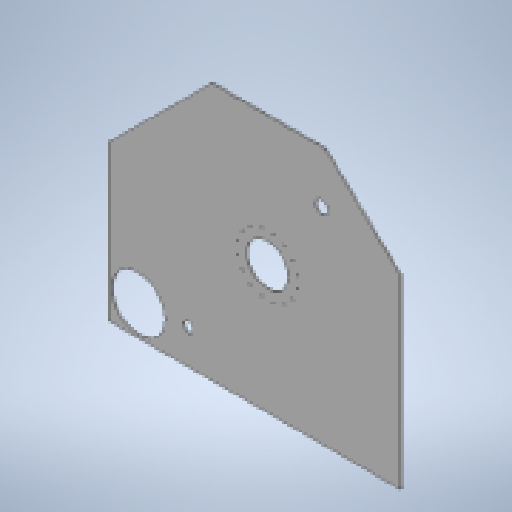
# Autodesk Inventor part: Left wall v2.0
Saved by Autodesk Inventor 2026.3 (Build 303398000, 398)
## iProperties
Created: 2023-08-31
Part Number: Left wall v2.0
Material: Generic
Document SubType Name: Sheet Metal
Designer: admin
Density: 1 g/cm^3
Appearance: Default
Flat Pattern Width: 191 cm
Flat Pattern Length: 217 cm
Flat Pattern Area: 41447 cm^2
Sheet Metal Rule: Default
Sheet Metal Width: 1910,000 mm
Sheet Metal Length: 2170,000 mm
Sheet Metal Area: 4144700,000 mm^2
Stock Number: ДМФ 013 Стенка Нос
Author: admin
Autodesk Inventor part; units mm, degrees
ref_plane "YZ Plane" through (0, 0, 0) normal (1, 0, 0) x (0, 1, 0)
ref_plane "XZ Plane" through (0, 0, 0) normal (0, 1, 0) x (-1, 0, 0)
ref_plane "XY Plane" through (0, 0, 0) normal (0, 0, 1) x (1, 0, 0)
sketch "Sketch1" plane through (0, 0, 0) normal (0, 0, 1) x (1, 0, 0)
  line L0 (519.5155, 1910) -> (-320.4845, 1910)
  line L1 (-320.4845, 1910) -> (-1085, 1150)
  line L2 (-1085, 0) -> (-1085, 1150)
  line L3 (1085, 0) -> (1085, 1372.7595)
  line L4 (519.5155, 1910) -> (1085, 1372.7595)
  line L5 (1085, 0) -> (-1085, 0)
  circle A0 centre (-865, 220) radius 200.5
  circle A1 centre (-493, 255) radius 38
  circle A2 centre (120, 955) radius 700 construction
  line L6 (499.31, 1277) -> (499.31, 1910) construction
  circle A3 centre (499.31, 1543.323) radius 30
  line L7 (1085, 955) -> (325, 955) construction
  circle A4 centre (120, 955) radius 205
  line L8 (120, 0) -> (120, 750) construction
  circle A5 centre (120, 955) radius 225 construction
  circle A6 centre (163.8953, 1175.6767) radius 6
  line L9 (120, 955) -> (120, 1180) construction
  line L10 (163.8953, 1175.6767) -> (120, 955) construction
  circle A7 centre (76.1047, 1175.6767) radius 6
  circle A8 centre (-5.0033, 1142.0807) radius 6
  circle A9 centre (-67.0807, 1080.0033) radius 6
  circle A10 centre (-100.6767, 998.8953) radius 6
  circle A11 centre (-100.6767, 911.1047) radius 6
  circle A12 centre (-67.0807, 829.9967) radius 6
  circle A13 centre (-5.0033, 767.9193) radius 6
  circle A14 centre (76.1047, 734.3233) radius 6
  circle A15 centre (163.8953, 734.3233) radius 6
  circle A16 centre (245.0033, 767.9193) radius 6
  circle A17 centre (307.0807, 829.9967) radius 6
  circle A18 centre (340.6767, 911.1047) radius 6
  circle A19 centre (340.6767, 998.8953) radius 6
  circle A20 centre (307.0807, 1080.0033) radius 6
  circle A21 centre (245.0033, 1142.0807) radius 6
  circle A22 centre (120, 955) radius 670 construction
  point P0 (0, 0)
  dimension "d69" = 1400
  dimension "d1" = 840
  dimension "d3" = 1150
  dimension "d14" = 76
  dimension "d15" = 1910
  dimension "d16" = 255
  dimension "d17" = 220
  dimension "d18" = 401
  dimension "d19" = 220
  dimension "d33" = 2170
  dimension "d49" = 372
  dimension "d51" = 780
  dimension "d52" = 1078
  dimension "d70" = 1584.31
  dimension "d71" = 60
  dimension "d74" = 760
  dimension "d75" = 410
  dimension "d76" = 750
  dimension "d77" = 450
  dimension "d78" = 12
  dimension "d79" = 11.25
  dimension "d82" = 360
  dimension "d84" = 465
  constraints: 22 centre point, 22 end point, 4 coincident, 4 point on circle, 4 point on line, 4 vertical, 2 horizontal, 2 line through centre, 2 midpoint, 1 perpendicular, 1 tangent, 36 other
  measures "d1" distance of L0.start L0.end
  measures "d3" distance of L2.start L1.end
  measures "d14" diameter of A1
  measures "d15" vertical distance of L2.start L0.end
  measures "d16" distance from line of A1.centre L5
  measures "d17" distance from line of L2 A0.centre
  measures "d18" diameter of A0
  measures "d19" distance from line of A0.centre L5
  measures "d33" distance of L3.start L2.start
  measures "d49" horizontal distance of A0.centre A1.centre
  measures "d51" distance of L0.start L3.end
  measures "d52" distance of L0.end L1.end
  measures "d70" distance between parallel lines of L2 L6
  measures "d71" diameter of A3
  measures "d74" distance of L7.start L7.end
  measures "d75" diameter of A4
  measures "d76" distance of L8.start L8.end
  measures "d77" diameter of A5
  measures "d78" diameter of A6
  measures "d79" angle of L9 L10
  measures "d84" radial gap between concentric circles of A4 A22
extrude "Extrusion5" add sketch "Sketch1" along normal blind 10
equation "\"d17\" = d19"
body "Solid2"
